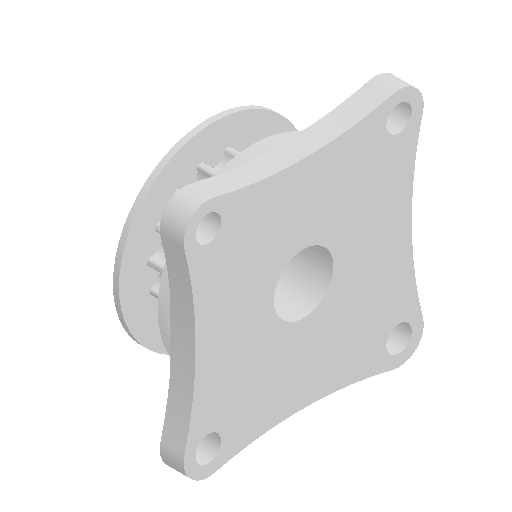
# Autodesk Inventor part: wheelBearingInside3.1
Saved by Autodesk Inventor 2023 (Build 270158000, 158)
## iProperties
Created: 2022-09-04
Part Number: wheelBearingInside3.1
Material: Generic
Document SubType Name: Modeling
Designer: deli
Density: 1 g/cm^3
Appearance: Default
Author: deli
Autodesk Inventor part; units mm, degrees
ref_plane "YZ Plane" through (0, 0, 0) normal (1, 0, 0) x (0, 1, 0)
ref_plane "XZ Plane" through (0, 0, 0) normal (0, 1, 0) x (-1, 0, 0)
sketch "Sketch1" plane through (0, 0, 0) normal (1, 0, 0) x (0, 1, 0)
  circle A0 centre (27.2703, 159.3312) radius 18
  circle A1 centre (27.2703, 159.3312) radius 5
  point P0 (0, 0)
  dimension "d0" = 36
  dimension "d6" = 10
  constraints: 2 centre point, 1 coincident
  measures "d0" diameter of A0
  measures "d6" diameter of A1
extrude "Extrusion1" add sketch "Sketch1" along normal blind 16
ref_plane "Work Plane1" through (8.5, 27.2703, 159.3312) normal (1, 0, 0) x (0, 0, -1)
sketch "Sketch4" plane through (8.5, 27.2703, 159.3312) normal (1, 0, 0) x (0, 0, -1)
  circle A0 centre (0, 0) radius 17.25 projected
  arc A1 (20.0191, 14.9661) -> (14.9661, 20.0191) centre (16, 16) ccw projected
  arc A2 (20.0191, 14.9661) -> (20.0191, -14.9661) centre (78.1974, 0) ccw projected
  arc A3 (14.9661, -20.0191) -> (20.0191, -14.9661) centre (16, -16) ccw projected
  arc A4 (14.9661, -20.0191) -> (-14.9661, -20.0191) centre (0, -78.1974) ccw projected
  arc A5 (-20.0191, -14.9661) -> (-14.9661, -20.0191) centre (-16, -16) ccw projected
  arc A6 (-20.0191, -14.9661) -> (-20.0191, 14.9661) centre (-78.1974, 0) ccw projected
  arc A7 (-14.9661, 20.0191) -> (-20.0191, 14.9661) centre (-16, 16) ccw projected
  arc A8 (-14.9661, 20.0191) -> (14.9661, 20.0191) centre (0, 78.1974) ccw projected
  circle A9 centre (-16, -16) radius 2.15 projected
  circle A10 centre (16, -16) radius 2.15 projected
  circle A11 centre (-16, 16) radius 2.15 projected
  circle A12 centre (16, 16) radius 2.15 projected
  point P0 (159.3312, -27.2703)
extrude "Extrusion4" add sketch "Sketch4" against normal blind 4
sketch "Sketch5" plane through (0, 27.2703, 159.3312) normal (-1, 0, 0) x (0, 0, 1)
  arc A0 (2.5155, 11.083) -> (2.2098, 11.1479) centre (0, 0) ccw projected
  arc A1 (2.2098, 11.1479) -> (1.7062, 10.8184) centre (2.1262, 10.7262) ccw projected
  line L0 (1.6959, 10.7713) -> (1.7062, 10.8184) projected
  arc A2 (0.359, 9.3598) -> (1.6959, 10.7713) centre (-0.1445, 11.1755) ccw projected
  arc A3 (0.359, 9.3598) -> (-0.359, 9.3598) centre (0, 0) ccw projected
  arc A4 (-1.6959, 10.7713) -> (-0.359, 9.3598) centre (0.1445, 11.1755) ccw projected
  line L1 (-1.6959, 10.7713) -> (-1.7062, 10.8184) projected
  arc A5 (-1.7062, 10.8184) -> (-2.2098, 11.1479) centre (-2.1262, 10.7262) ccw projected
  arc A6 (-2.2098, 11.1479) -> (-2.5155, 11.083) centre (0, 0) ccw projected
  arc A7 (-2.5155, 11.083) -> (-2.8415, 10.5771) centre (-2.4203, 10.6636) ccw projected
  line L2 (-2.8318, 10.5298) -> (-2.8415, 10.5771) projected
  arc A8 (-3.479, 8.6966) -> (-2.8318, 10.5298) centre (-4.6775, 10.1505) ccw projected
  arc A9 (-3.479, 8.6966) -> (-4.1349, 8.4046) centre (0, 0) ccw projected
  arc A10 (-5.9303, 9.1503) -> (-4.1349, 8.4046) centre (-4.4135, 10.2681) ccw projected
  line L3 (-5.9303, 9.1503) -> (-5.9589, 9.1891) projected
  arc A11 (-5.9589, 9.1891) -> (-6.553, 9.2853) centre (-6.3051, 8.934) ccw projected
  arc A12 (-6.553, 9.2853) -> (-6.8059, 9.1016) centre (0, 0) ccw projected
  arc A13 (-6.8059, 9.1016) -> (-6.898, 8.5069) centre (-6.5484, 8.7573) ccw projected
  line L4 (-6.8699, 8.4677) -> (-6.898, 8.5069) projected
  arc A14 (-6.7154, 6.5297) -> (-6.8699, 8.4677) centre (-8.4017, 7.3705) ccw projected
  arc A15 (-6.7154, 6.5297) -> (-7.1959, 5.9961) centre (0, 0) ccw projected
  arc A16 (-9.1394, 5.9471) -> (-7.1959, 5.9961) centre (-8.2083, 7.5852) ccw projected
  line L5 (-9.1394, 5.9471) -> (-9.1813, 5.971) projected
  arc A17 (-9.1813, 5.971) -> (-9.7632, 5.8172) centre (-9.3938, 5.5971) ccw projected
  arc A18 (-9.7632, 5.8172) -> (-9.9195, 5.5466) centre (0, 0) ccw projected
  arc A19 (-9.9195, 5.5466) -> (-9.7617, 4.9658) centre (-9.5441, 5.3367) ccw projected
  line L6 (-9.72, 4.9414) -> (-9.7617, 4.9658) projected
  arc A20 (-8.7907, 3.2338) -> (-9.72, 4.9414) centre (-10.6732, 3.316) ccw projected
  arc A21 (-8.7907, 3.2338) -> (-9.0126, 2.5509) centre (0, 0) ccw projected
  arc A22 (-10.7681, 1.7156) -> (-9.0126, 2.5509) centre (-10.5839, 3.5908) ccw projected
  line L7 (-10.7681, 1.7156) -> (-10.8162, 1.7204) projected
  arc A23 (-10.8162, 1.7204) -> (-11.2852, 1.3432) centre (-10.8582, 1.2924) ccw projected
  arc A24 (-11.2852, 1.3432) -> (-11.3179, 1.0324) centre (0, 0) ccw projected
  arc A25 (-11.3179, 1.0324) -> (-10.9375, 0.566) centre (-10.8896, 0.9934) ccw projected
  line L8 (-10.8895, 0.5607) -> (-10.9375, 0.566) projected
  arc A26 (-9.346, -0.6213) -> (-10.8895, 0.5607) centre (-11.0991, -1.3118) ccw projected
  arc A27 (-9.346, -0.6213) -> (-9.271, -1.3354) centre (0, 0) ccw projected
  arc A28 (-10.535, -2.8125) -> (-9.271, -1.3354) centre (-11.1294, -1.0245) ccw projected
  line L9 (-10.535, -2.8125) -> (-10.5808, -2.8277) projected
  arc A29 (-10.5808, -2.8277) -> (-10.8559, -3.363) centre (-10.4451, -3.2357) ccw projected
  arc A30 (-10.8559, -3.363) -> (-10.7593, -3.6602) centre (0, 0) ccw projected
  arc A31 (-10.7593, -3.6602) -> (-10.2221, -3.9316) centre (-10.3522, -3.5217) ccw projected
  line L10 (-10.1761, -3.917) -> (-10.2221, -3.9316) projected
  arc A32 (-8.2853, -4.369) -> (-10.1761, -3.917) centre (-9.606, -5.7129) ccw projected
  arc A33 (-8.2853, -4.369) -> (-7.9263, -4.9908) centre (0, 0) ccw projected
  arc A34 (-8.4803, -6.8543) -> (-7.9263, -4.9908) centre (-9.7505, -5.4626) ccw projected
  line L11 (-8.4803, -6.8543) -> (-8.5159, -6.8868) projected
  arc A35 (-8.5159, -6.8868) -> (-8.5495, -7.4877) centre (-8.226, -7.2044) ccw projected
  arc A36 (-8.5495, -7.4877) -> (-8.3404, -7.72) centre (0, 0) ccw projected
  arc A37 (-8.3404, -7.72) -> (-7.7392, -7.7494) centre (-8.0248, -7.4279) ccw projected
  line L12 (-7.7032, -7.7173) -> (-7.7392, -7.7494) projected
  arc A38 (-5.792, -7.3612) -> (-7.7032, -7.7173) centre (-6.4519, -9.1261) ccw projected
  arc A39 (-5.792, -7.3612) -> (-5.2111, -7.7832) centre (0, 0) ccw projected
  arc A40 (-4.9592, -9.7109) -> (-5.2111, -7.7832) centre (-6.6857, -8.9562) ccw projected
  line L13 (-4.9592, -9.7109) -> (-4.9785, -9.7552) projected
  arc A41 (-4.9785, -9.7552) -> (-4.7648, -10.3178) centre (-4.5845, -9.9274) ccw projected
  arc A42 (-4.7648, -10.3178) -> (-4.4793, -10.4449) centre (0, 0) ccw projected
  arc A43 (-4.4793, -10.4449) -> (-3.9182, -10.2272) centre (-4.3098, -10.0497) ccw projected
  line L14 (-3.8983, -10.1833) -> (-3.9182, -10.2272) projected
  arc A44 (-2.2972, -9.0806) -> (-3.8983, -10.1833) centre (-2.1822, -10.9613) ccw projected
  arc A45 (-2.2972, -9.0806) -> (-1.5948, -9.2299) centre (0, 0) ccw projected
  arc A46 (-0.5807, -10.8885) -> (-1.5948, -9.2299) centre (-2.4648, -10.9012) ccw projected
  line L15 (-0.5807, -10.8885) -> (-0.5803, -10.9367) projected
  arc A47 (-0.5803, -10.9367) -> (-0.1563, -11.3638) centre (-0.1504, -10.9338) ccw projected
  arc A48 (-0.1563, -11.3638) -> (0.1563, -11.3638) centre (0, 0) ccw projected
  arc A49 (0.1563, -11.3638) -> (0.5803, -10.9367) centre (0.1504, -10.9338) ccw projected
  line L16 (0.5807, -10.8885) -> (0.5803, -10.9367) projected
  arc A50 (1.5948, -9.2299) -> (0.5807, -10.8885) centre (2.4648, -10.9012) ccw projected
  arc A51 (1.5948, -9.2299) -> (2.2972, -9.0806) centre (0, 0) ccw projected
  arc A52 (3.8983, -10.1833) -> (2.2972, -9.0806) centre (2.1822, -10.9613) ccw projected
  line L17 (3.8983, -10.1833) -> (3.9182, -10.2272) projected
  arc A53 (3.9182, -10.2272) -> (4.4793, -10.4449) centre (4.3098, -10.0497) ccw projected
  arc A54 (4.4793, -10.4449) -> (4.7648, -10.3178) centre (0, 0) ccw projected
  arc A55 (4.7648, -10.3178) -> (4.9785, -9.7552) centre (4.5845, -9.9274) ccw projected
  line L18 (4.9592, -9.7109) -> (4.9785, -9.7552) projected
  arc A56 (5.2111, -7.7832) -> (4.9592, -9.7109) centre (6.6857, -8.9562) ccw projected
  arc A57 (5.2111, -7.7832) -> (5.792, -7.3612) centre (0, 0) ccw projected
  arc A58 (7.7032, -7.7173) -> (5.792, -7.3612) centre (6.4519, -9.1261) ccw projected
  line L19 (7.7032, -7.7173) -> (7.7392, -7.7494) projected
  arc A59 (7.7392, -7.7494) -> (8.3404, -7.72) centre (8.0248, -7.4279) ccw projected
  arc A60 (8.3404, -7.72) -> (8.5495, -7.4877) centre (0, 0) ccw projected
  arc A61 (8.5495, -7.4877) -> (8.5159, -6.8868) centre (8.226, -7.2044) ccw projected
  line L20 (8.4803, -6.8543) -> (8.5159, -6.8868) projected
  arc A62 (7.9263, -4.9908) -> (8.4803, -6.8543) centre (9.7505, -5.4626) ccw projected
  arc A63 (7.9263, -4.9908) -> (8.2853, -4.369) centre (0, 0) ccw projected
  arc A64 (10.1761, -3.917) -> (8.2853, -4.369) centre (9.606, -5.7129) ccw projected
  line L21 (10.1761, -3.917) -> (10.2221, -3.9316) projected
  arc A65 (10.2221, -3.9316) -> (10.7593, -3.6602) centre (10.3522, -3.5217) ccw projected
  arc A66 (10.7593, -3.6602) -> (10.8559, -3.363) centre (0, 0) ccw projected
  arc A67 (10.8559, -3.363) -> (10.5808, -2.8277) centre (10.4451, -3.2357) ccw projected
  line L22 (10.535, -2.8125) -> (10.5808, -2.8277) projected
  arc A68 (9.271, -1.3354) -> (10.535, -2.8125) centre (11.1294, -1.0245) ccw projected
  arc A69 (9.271, -1.3354) -> (9.346, -0.6213) centre (0, 0) ccw projected
  arc A70 (10.8895, 0.5607) -> (9.346, -0.6213) centre (11.0991, -1.3118) ccw projected
  line L23 (10.8895, 0.5607) -> (10.9375, 0.566) projected
  arc A71 (10.9375, 0.566) -> (11.3179, 1.0324) centre (10.8896, 0.9934) ccw projected
  arc A72 (11.3179, 1.0324) -> (11.2852, 1.3432) centre (0, 0) ccw projected
  arc A73 (11.2852, 1.3432) -> (10.8162, 1.7204) centre (10.8582, 1.2924) ccw projected
  line L24 (10.7681, 1.7156) -> (10.8162, 1.7204) projected
  arc A74 (9.0126, 2.5509) -> (10.7681, 1.7156) centre (10.5839, 3.5908) ccw projected
  arc A75 (9.0126, 2.5509) -> (8.7907, 3.2338) centre (0, 0) ccw projected
  arc A76 (9.72, 4.9414) -> (8.7907, 3.2338) centre (10.6732, 3.316) ccw projected
  line L25 (9.72, 4.9414) -> (9.7617, 4.9658) projected
  arc A77 (9.7617, 4.9658) -> (9.9195, 5.5466) centre (9.5441, 5.3367) ccw projected
  arc A78 (9.9195, 5.5466) -> (9.7632, 5.8172) centre (0, 0) ccw projected
  arc A79 (9.7632, 5.8172) -> (9.1813, 5.971) centre (9.3938, 5.5971) ccw projected
  line L26 (9.1394, 5.9471) -> (9.1813, 5.971) projected
  arc A80 (7.1959, 5.9961) -> (9.1394, 5.9471) centre (8.2083, 7.5852) ccw projected
  arc A81 (7.1959, 5.9961) -> (6.7154, 6.5297) centre (0, 0) ccw projected
  arc A82 (6.8699, 8.4677) -> (6.7154, 6.5297) centre (8.4017, 7.3705) ccw projected
  line L27 (6.8699, 8.4677) -> (6.898, 8.5069) projected
  arc A83 (6.898, 8.5069) -> (6.8059, 9.1016) centre (6.5484, 8.7573) ccw projected
  arc A84 (6.8059, 9.1016) -> (6.553, 9.2853) centre (0, 0) ccw projected
  arc A85 (6.553, 9.2853) -> (5.9589, 9.1891) centre (6.3051, 8.934) ccw projected
  line L28 (5.9303, 9.1503) -> (5.9589, 9.1891) projected
  arc A86 (4.1349, 8.4046) -> (5.9303, 9.1503) centre (4.4135, 10.2681) ccw projected
  arc A87 (4.1349, 8.4046) -> (3.479, 8.6966) centre (0, 0) ccw projected
  arc A88 (2.8318, 10.5298) -> (3.479, 8.6966) centre (4.6775, 10.1505) ccw projected
  line L29 (2.8318, 10.5298) -> (2.8415, 10.5771) projected
  arc A89 (2.8415, 10.5771) -> (2.5155, 11.083) centre (2.4203, 10.6636) ccw projected
  circle A90 centre (0, 0) radius 5 projected
  point P0 (-159.3312, -27.2703)
extrude "Extrusion5" add sketch "Sketch5" along normal blind 6.5
chamfer "Chamfer1" distance 4.5 distance2 2 1 edges at (0, 9.2703, 159.3312) measured on face at (0.5, 9.2703, 159.3312)
fillet "Fillet1" radius 2 2 edges at (4.4999, 9.2703, 159.3312) (4.5, 9.2703, 159.3312)
sketch "Sketch6" plane through (-6.5, 27.2703, 159.3312) normal (-1, 0, 0) x (0, 0, 1)
  circle A0 centre (0, 0) radius 16 projected
  circle A1 centre (0, 0) radius 5 projected
  point P0 (-159.3312, -27.2703)
extrude "Extrusion6" add sketch "Sketch6" along normal blind 1
sketch "Sketch7" plane through (8.5, 27.2703, 159.3312) normal (1, 0, 0) x (0, 0, -1)
  line L0 (-25.5923, 21.2252) -> (27.7289, 21.2252)
  line L1 (27.7289, 21.2252) -> (27.7289, -27.2703)
  line L2 (27.7289, -27.2703) -> (-25.5923, -27.2703)
  line L3 (-25.5923, -27.2703) -> (-25.5923, 21.2252)
  point P0 (159.3312, -27.2703)
  constraints: 8 end point, 2 parallel, 1 horizontal, 1 perpendicular
extrude "Extrusion7" cut sketch "Sketch7" along normal blind 10
sketch "Sketch8" plane through (-7.5, 27.2703, 159.3312) normal (-1, 0, 0) x (0, 0, 1)
  circle A0 centre (0, 0) radius 7
  point P0 (-159.3312, -27.2703)
  dimension "d26" = 14
  constraints: 1 centre point
  measures "d26" diameter of A0
extrude "Extrusion8" cut sketch "Sketch8" against normal blind 5
sketch "Sketch9" plane through (-7.5, 27.2703, 159.3312) normal (-1, 0, 0) x (0, 0, 1)
  circle A0 centre (0, 0) radius 7.5
  point P0 (-159.3312, -27.2703)
  dimension "d29" = 15
  constraints: 1 centre point
  measures "d29" diameter of A0
extrude "Extrusion9" cut sketch "Sketch9" against normal blind 1
body "Solid1"
